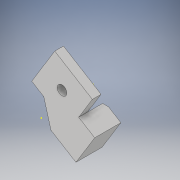
# Autodesk Inventor part: thumb_phalanx_plate
Saved by Autodesk Inventor 2019 (Build 230136000, 136)
## iProperties
Created: 2024-08-27
Part Number: thumb_phalanx_plate
Material: Generisch
Document SubType Name: Modeling
Designer: nic
Density: 1 g/cm^3
Appearance: Vorgabe
Author: nic
Autodesk Inventor part; units mm, degrees
ref_plane "YZ Plane" through (0, 0, 0) normal (1, 0, 0) x (0, 1, 0)
ref_plane "XZ Plane" through (0, 0, 0) normal (0, 1, 0) x (-1, 0, 0)
ref_plane "XY Plane" through (0, 0, 0) normal (0, 0, 1) x (1, 0, 0)
sketch "Skizze1" plane through (0, 0, 0) normal (0, 0, 1) x (1, 0, 0)
  circle A0 centre (11.2246, 18.4558) radius 0.3325 construction
  circle A1 centre (11.2246, 18.4558) radius 1.1
  circle A2 centre (11.2246, 18.4558) radius 2.5
  point P0 (0, 0)
  dimension "d0" = 2.2
  dimension "d1" = 5
  constraints: 2 centre point, 2 coincident
  measures "d0" diameter of A1
  measures "d1" diameter of A2
ref_plane "Arbeitsebene1" through (-2.597, -2.44, -3) normal (0, 0, -1) x (0, 1, 0)
extrude "Extrusion1" add sketch "Skizze1" against normal up to surface (3 mm away)
sketch "Skizze2" plane through (11.2246, 18.4558, 0) normal (0, 0, 1) x (1, 0, 0)
  line L0 (0, 0) -> (-2.8913, -4.716) construction
  line L1 (-2.8913, -4.716) -> (3.5184, 5.7389) construction
  line L2 (0, 0) -> (3.8461, -2.358) construction
  line L3 (-6.9448, -1.6658) -> (-1.6658, 6.9448)
  line L4 (-1.6658, 6.9448) -> (6.9448, 1.6658)
  line L5 (6.9448, 1.6658) -> (1.6658, -6.9448)
  line L6 (1.6658, -6.9448) -> (-6.9448, -1.6658)
  line L7 (-6.9448, -1.6658) -> (6.9448, 1.6658) construction
  line L8 (-1.6658, 6.9448) -> (1.6658, -6.9448) construction
  point P0 (-11.2246, -18.4558)
  dimension "d4" = 10.1
  dimension "d5" = 10.1
  constraints: 18 end point, 2 midpoint, 2 parallel, 2 perpendicular, 1 point on line
  measures "d4" distance of L3.start L3.end
  measures "d5" distance of L3.end L4.end
extrude "Extrusion2" add sketch "Skizze2" against normal blind 2
sketch "Skizze3" plane through (0, 0, 0) normal (0, 0, 1) x (1, 0, 0)
  line L0 (4.2798, 16.79) -> (9.5588, 25.4006) projected
  line L1 (12.8904, 11.511) -> (4.2798, 16.79) projected
  line L2 (18.1694, 20.1216) -> (12.8904, 11.511) projected
  line L3 (9.5588, 25.4006) -> (18.1694, 20.1216) projected
  line L4 (4.8948, 11.5894) -> (14.4118, 5.7548)
  line L5 (14.4118, 5.7548) -> (18.7104, 12.7664)
  line L6 (18.7104, 12.7664) -> (15.0398, 15.0168)
  line L7 (-1.5402, 15.5346) -> (18.7104, 12.7664) construction
  line L8 (14.4118, 5.7548) -> (2.7585, 22.5462) construction
  line L9 (4.8948, 11.5894) -> (7.0442, 15.0952)
  line L10 (12.8904, 11.511) -> (4.2798, 16.79) projected
  line L11 (7.0442, 15.0952) -> (12.8904, 11.511)
  line L12 (12.8904, 11.511) -> (15.0398, 15.0168)
  line L13 (18.1694, 20.1216) -> (12.8904, 11.511) projected
  point P0 (0, 0)
  point P1 (8.5851, 14.1505)
  constraints: 16 end point, 3 midpoint, 2 perpendicular, 2 point on line, 1 parallel
extrude "Extrusion3" add sketch "Skizze3" against normal blind 6 contours L1 L2 L6 L5 L4 L9
sketch "Skizze4" plane through (4.8948, 11.5894, -6) normal (-0.5226725, -0.8525335, 0) x (0.8525335, -0.5226725, 0)
  line L0 (-1.036, 2.1441) -> (1.7865, 3.0085) projected
  line L1 (0, 6) -> (11.1631, 6) projected
  line L2 (0, 6) -> (0, 0) projected
  line L3 (11.1631, 0) -> (0, 0) projected
  line L4 (11.1631, 6) -> (11.1631, 0) projected
  line L5 (0.7075, 3) -> (2.9075, 3) projected
  line L6 (1.3376, -2.7865) -> (1.3376, -9.7615) projected
  ellipse E0 centre (1.3376, -6.274) end of major axis (1.3376, 3) minor radius 7.5665
  point P0 (1.8845, 6)
  constraints: 1 horizontal, 1 midpoint, 2 other
extrude "Extrusion4" cut sketch "Skizze4" against normal up to surface (8.2244 mm away) contours L2 E0 L0 | L2 L3 E0 | L0 E0 L3 L2
sketch "Skizze5" plane through (0, 0, 0) normal (0, 0, 1) x (1, 0, 0)
  line L0 (4.2798, 16.79) -> (9.5588, 25.4006) projected
  line L1 (7.0442, 15.0952) -> (4.2798, 16.79) projected
  line L2 (7.0442, 15.0952) -> (4.8948, 11.5894) projected
  line L3 (4.8948, 11.5894) -> (14.4118, 5.7548) projected
  line L4 (14.4118, 5.7548) -> (18.7104, 12.7664) projected
  line L5 (18.7104, 12.7664) -> (15.0398, 15.0168) projected
  line L6 (18.1694, 20.1216) -> (15.0398, 15.0168) projected
  line L7 (9.5588, 25.4006) -> (18.1694, 20.1216) projected
  line L8 (7.0442, 15.0952) -> (4.8948, 11.5894) projected
  line L9 (7.0442, 15.0952) -> (8.6934, 9.2606)
  line L10 (10.7856, 7.9779) -> (4.8948, 11.5894) projected
  point P0 (0, 0)
  constraints: 2 end point, 1 point on line
extrude "Extrusion5" cut sketch "Skizze5" against normal blind 6 contours L9 L3 L2
chamfer "Fase1" distance 1 angle 45 1 edges at (12.9349, 11.4837, -6)
sketch "Skizze6" plane through (14.4118, 5.7548, -6) normal (-0.5226725, -0.8525335, 0) x (0.8525335, -0.5226725, 0)
  ellipse E0 centre (-9.8255, -6.274) end of major axis (-9.8255, -15.548) minor radius 7.5665 (-4.8984, 0.7642) -> (-6.7074, 2.1759) ccw projected
  ellipse E1 centre (-9.8255, -6.274) end of major axis (-9.8255, -15.548) minor radius 7.5665 (-6.7074, 2.1759) -> (-11.1631, 2.8539) ccw projected
  point P0 (-9.2786, 6)
  constraints: 3 other
sketch "Skizze7" plane through (11.2246, 18.4558, -3) normal (0, 0, -1) x (-1, 0, 0)
  circle A0 centre (0, 0) radius 1.1 projected
  point P0 (11.2246, -18.4558)
extrude "Extrusion6" cut sketch "Skizze7" against normal blind 10
